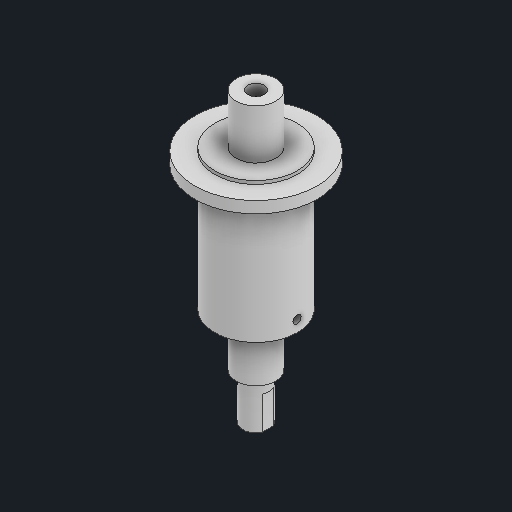
# Autodesk Inventor part: shaft
Saved by Autodesk Inventor 2025.2 (Build 292293000, 293)
## iProperties
Created: 2025-04-19
Part Number: shaft
Material: Generic
Document SubType Name: Modeling
Designer: klawy
Density: 1 g/cm^3
Appearance: Default
Mass: 21.1173 g
Surface Area: 80.0172 cm^2
Volume: 21.1173 cm^3
Author: klawy
Autodesk Inventor part; units mm, degrees
ref_plane "XZ Plane" through (0, 0, 0) normal (0, 1, 0) x (-1, 0, 0)
ref_plane "XY Plane" through (0, 0, 0) normal (0, 0, 1) x (1, 0, 0)
sketch "Sketch1" plane through (0, 0, 0) normal (0, 0, 1) x (1, 0, 0)
  line L0 (0, -17.5) -> (8.5, -17.5)
  line L1 (8.5, -17.5) -> (8.5, 17.5)
  line L2 (8.5, 17.5) -> (0, 17.5)
  line L3 (0, 17.5) -> (0, -17.5)
  line L4 (8.5, 11.5) -> (18.5, 11.5)
  line L5 (18.5, 11.5) -> (18.5, 9)
  line L6 (18.5, 9) -> (8.5, 9)
  line L7 (8.5, 9) -> (8.5, 11.5)
  line L8 (18.5, 9) -> (15.5, 9)
  line L9 (15.5, 9) -> (15.5, 8)
  line L10 (15.5, 8) -> (18.5, 8)
  line L11 (18.5, 8) -> (18.5, 9)
  line L12 (0, -24.5) -> (0, 24.5) construction
  line L13 (8.5, -17.5) -> (12.5, -17.5)
  line L14 (12.5, -17.5) -> (12.5, 9)
  line L15 (12.5, 9) -> (8.5, 9)
  line L16 (8.5, 9) -> (8.5, -17.5)
  line L17 (8.5, 11.5) -> (6, 11.5)
  line L18 (6, 11.5) -> (6, 17.5)
  point P0 (0, 0)
  point P1 (0, 0)
  point P2 (8.5, 9)
  dimension "d0" = 35
  dimension "d1" = 8.5
  dimension "d2" = 10
  dimension "d3" = 2.5
  dimension "d4" = 6
  dimension "d5" = 3
  dimension "d6" = 1
  dimension "d32" = 4
  dimension "d69" = 6
  constraints: 36 end point, 8 parallel, 5 horizontal, 5 perpendicular, 3 point on line, 2 coincident, 1 midpoint
  measures "d0" distance of L0.end L1.end
  measures "d1" distance of L1.end L2.end
  measures "d2" distance between parallel lines of L1 L5
  measures "d3" distance between parallel lines of L4 L6
  measures "d4" distance between parallel lines of L2 L4
  measures "d5" distance between parallel lines of L11 L9
  measures "d6" distance from line of L5.end L10
  measures "d32" distance between parallel lines of L1 L14
  measures "d69" distance between parallel lines of L18 L3
revolve "Revolution1" add sketch "Sketch1" angle 360 about axis through (0, -10, 0) along (0, 1, 0) contours L3 L2 L18 L17 L1 L0 | L1 L6 L14 L13 | L1 L4 L5 L6 | L6 L11 L10 L9
sketch "Sketch3" plane through (0, -17.5, 0) normal (0, -1, 0) x (1, 0, 0)
  circle A0 centre (0, 0) radius 12.5 projected
extrude "Extrusion1" add sketch "Sketch3" along normal blind 12.5
sketch "Sketch4" plane through (0, -30, 0) normal (0, -1, 0) x (1, 0, 0)
  circle A0 centre (0, 0) radius 4
  circle A1 centre (0, 0) radius 12.5 projected
  dimension "d24" = 8
  constraints: 2 coincident, 1 centre point
  measures "d24" diameter of A0
extrude "Extrusion2" add sketch "Sketch4" along normal blind 29.75 contours A0
sketch "Sketch5" plane through (0, 17.5, 0) normal (0, 1, 0) x (1, 0, 0)
  circle A0 centre (0, 0) radius 6 projected
extrude "Extrusion3" add sketch "Sketch5" along normal blind 10
sketch "Sketch6" plane through (0, 11.5, 0) normal (0, 1, 0) x (1, 0, 0)
  circle A0 centre (0, 0) radius 2.621 projected
  circle A1 centre (0, 0) radius 12.5
  circle A2 centre (0, 0) radius 6 projected
  dimension "d29" = 25
  constraints: 1 centre point, 1 coincident
  measures "d29" diameter of A1
extrude "Extrusion4" add sketch "Sketch6" along normal blind 1 contours A0 | A1 | A2
sketch "Sketch7" plane through (0, 27.5, 0) normal (0, 1, 0) x (1, 0, 0)
  point P0 (0, 0)
  point P1 (0, 0)
  constraints: 1 coincident
hole "Hole2" at (0, 27.5, 0) direction (0, -1, 0) diameter 3.242 end through all thread size "M4x0.7" class "6H" standard "ISO Metric profile"
sketch "Sketch8" plane through (0, 27.5, 0) normal (0, 1, 0) x (1, 0, 0)
  circle A0 centre (0, 0) radius 2.5
  dimension "d41" = 5
  constraints: 1 centre point, 1 coincident
  measures "d41" diameter of A0
extrude "Extrusion5" cut sketch "Sketch8" against normal blind 10
sketch "Sketch9" plane through (0, -59.75, 0) normal (0, -1, 0) x (1, 0, 0)
  circle A0 centre (0, 0) radius 2.5
  dimension "d44" = 5
  constraints: 1 centre point, 1 coincident
  measures "d44" diameter of A0
extrude "Extrusion6" cut sketch "Sketch9" against normal blind 50
chamfer "Chamfer3" distance 0.5 angle 30 1 edges at (0, -9.75, -1.621) measured on face at (2.1788, -9.75, -0.2646)
chamfer "Chamfer4" distance 0.5 angle 30 1 edges at (0, 17.5, -1.621) measured on face at (2.1788, 17.5, 0.2646)
ref_plane "Work Plane1" through (12.5, 0, 0) normal (1, 0, 0) x (0, 1, 0)
sketch "Sketch10" plane through (12.5, 0, 0) normal (1, 0, 0) x (0, 1, 0)
  line L0 (27.5, -8.5) -> (27.5, 8.5) projected
  line L1 (-37.3, 0) -> (38.3, 0) projected
  point P0 (0, 0)
  point P1 (-26.5, 0)
  dimension "d54" = 54
  constraints: 1 point on line
  measures "d54" distance from line of point (-26.5, 0) L0
hole "Hole3" at (12.5, -26.5, 0) direction (-1, 0, 0) diameter 2.459 depth 8.8 tip angle 118 thread size "M3x0.5" class "6H" standard "ISO Metric profile"
sketch "Sketch11" plane through (0, -59.75, 0) normal (0, -1, 0) x (1, 0, 0)
  circle A0 centre (0, 0) radius 2.5 projected
  circle A1 centre (0, 0) radius 4 projected
  line L0 (3.6, -1.7436) -> (3.6, 1.7436)
  point P0 (3.6, 0)
  dimension "d65" = 3.6
  constraints: 2 end point, 2 point on circle, 1 midpoint, 1 vertical
  measures "d65" distance from line of L0 point (0, 0)
extrude "Extrusion7" cut sketch "Sketch11" against normal blind 10 contours A0 | A1 L0 picked at (3.6735, -0.3949)
sketch "Sketch12" plane through (0, -30, 0) normal (0, -1, 0) x (1, 0, 0)
  circle A0 centre (0, 0) radius 6
  circle A1 centre (0, 0) radius 2.5 projected
  dimension "d66" = 12
  constraints: 1 centre point, 1 coincident
  measures "d66" diameter of A0
extrude "Extrusion8" add sketch "Sketch12" along normal blind 16
body "Solid1"
